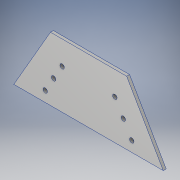
# Autodesk Inventor part: nhk22
Saved by Autodesk Inventor 2019 (Build 230136000, 136)
## iProperties
Created: 2022-02-15
Part Number: nhk22
Material: アルミニウム 6061
Document SubType Name: Sheet Metal
Designer: yuta
Density: 2.7 g/cm^3
Sheet Metal Rule: Default_mm
Appearance: アルミニウム - フラット
Author: yuta
Autodesk Inventor part; units mm, degrees
ref_plane "YZ Plane" through (0, 0, 0) normal (1, 0, 0) x (0, 1, 0)
ref_plane "XZ Plane" through (0, 0, 0) normal (0, 1, 0) x (-1, 0, 0)
ref_plane "XY Plane" through (0, 0, 0) normal (0, 0, 1) x (1, 0, 0)
sketch "スケッチ1" plane through (0, 0, 0) normal (0, 0, 1) x (1, 0, 0)
  line L0 (-21.0154, -61.075) -> (70.9846, -61.075)
  line L1 (70.9846, -61.075) -> (50.9846, -26.434)
  line L2 (50.9846, -26.434) -> (-1.0154, -26.434)
  line L3 (-1.0154, -26.434) -> (-21.0154, -61.075)
  point P0 (0, 0)
  dimension "d0" = 92
  dimension "d1" = 40
  dimension "d2" = 60
  dimension "d3" = 52
  constraints: 8 end point, 1 horizontal, 1 parallel
  measures "d0" distance of L0.start L0.end
  measures "d1" distance of L0.end L1.end
  measures "d2" angle of L1 L0
  measures "d3" distance of L1.end L2.end
extrude "押し出し1" add sketch "スケッチ1" along normal blind 2
sketch "スケッチ2" plane through (0, 0, 2) normal (0, 0, 1) x (1, 0, 0)
  circle A0 centre (6.975, -42.5942) radius 1.5
  line L0 (-1.0154, -26.434) -> (-21.0154, -61.075) projected
  line L1 (50.9846, -26.434) -> (-1.0154, -26.434) projected
  line L2 (-1.0154, -26.434) -> (24.9653, -41.434)
  line L3 (-1.0154, -26.434) -> (28.9846, -26.434) construction
  line L4 (70.9846, -61.075) -> (50.9846, -26.434) projected
  line L5 (50.9846, -26.434) -> (24.9751, -41.4506)
  circle A1 centre (1.2015, -52.5942) radius 1.5
  circle A2 centre (-4.572, -62.5942) radius 1.5
  line L6 (-21.0154, -61.075) -> (70.9846, -61.075) projected
  line L7 (-21.0154, -61.075) -> (-26.0154, -69.7352)
  line L8 (-21.0154, -61.075) -> (-11.0154, -61.075) construction
  line L9 (-26.0154, -69.7352) -> (75.9846, -69.7352)
  line L10 (75.9846, -69.7352) -> (70.9846, -61.075)
  point P0 (0, 0)
  dimension "d6" = 3
  dimension "d7" = 15
  dimension "d8" = 30
  dimension "d9" = 30
  dimension "d10" = 10
  dimension "d11" = 3
  dimension "d12" = 3
  dimension "d13" = 10
  dimension "d14" = 15
  dimension "d15" = 10
  dimension "d16" = 120
  dimension "d17" = 60
  dimension "d18" = 10
  dimension "d19" = 15
  constraints: 14 end point, 3 centre point, 2 equal length, 2 horizontal, 1 collinear, 1 perpendicular
  measures "d6" diameter of A0
  measures "d7" distance from line of L0 A0.centre
  measures "d8" distance of L0.start L2.end
  measures "d9" angle of L2 L3
  measures "d10" distance from line of L2 A0.centre
  measures "d11" diameter of A1
  measures "d12" diameter of A2
  measures "d13" vertical distance of A0.centre A1.centre
  measures "d14" distance from line of L0 A1.centre
  measures "d15" distance of L0.end L7.end
  measures "d16" angle of L7 L8
  measures "d17" angle of L9 L7
  measures "d18" vertical distance of A1.centre A2.centre
  measures "d19" distance from line of L0 A2.centre
extrude "押し出し2" add sketch "スケッチ2" against normal blind 2 contours L6 L10 L9 L7
sketch "スケッチ3" plane through (0, 0, 2) normal (0, 0, 1) x (1, 0, 0)
  line L0 (-1.0154, -26.434) -> (-26.0154, -69.7352) projected
  line L1 (-1.0154, -26.434) -> (24.9653, -41.434)
  line L2 (-1.0154, -26.434) -> (28.9846, -26.434) construction
  line L3 (24.9653, -41.434) -> (50.9461, -26.434)
  circle A0 centre (6.975, -42.5942) radius 1.5
  circle A1 centre (1.2015, -52.5942) radius 1.5
  circle A2 centre (42.9846, -42.5776) radius 1.5
  circle A3 centre (48.7581, -52.5776) radius 1.5
  circle A4 centre (54.5316, -62.5776) radius 1.5
  line L4 (75.9846, -69.7352) -> (50.9846, -26.434) projected
  point P0 (0, 0)
  dimension "d22" = 30
  dimension "d23" = 30
  dimension "d24" = 120
  dimension "d25" = 3
  dimension "d26" = 15
  dimension "d27" = 10
  dimension "d28" = 3
  dimension "d29" = 15
  dimension "d30" = 10
  dimension "d31" = 3
  dimension "d32" = 3
  dimension "d33" = 3
  dimension "d34" = 15
  dimension "d35" = 15
  dimension "d36" = 15
  dimension "d37" = 10
  dimension "d38" = 10
  dimension "d39" = 10
  constraints: 6 end point, 5 centre point, 1 equal length, 1 horizontal, 1 perpendicular
  measures "d22" distance of L0.start L1.end
  measures "d23" angle of L1 L2
  measures "d24" angle of L3 L1
  measures "d25" diameter of A0
  measures "d26" distance from line of L0 A0.centre
  measures "d27" distance from line of L1 A0.centre
  measures "d28" diameter of A1
  measures "d29" distance from line of L0 A1.centre
  measures "d30" vertical distance of A1.centre A0.centre
  measures "d31" diameter of A2
  measures "d32" diameter of A3
  measures "d33" diameter of A4
  measures "d34" distance from line of A2.centre L4
  measures "d35" distance from line of L4 A3.centre
  measures "d36" distance from line of L4 A4.centre
  measures "d37" distance from line of L3 A2.centre
  measures "d38" vertical distance of A3.centre A2.centre
  measures "d39" vertical distance of A4.centre A3.centre
hole "穴1" at (1.2015, -52.5942, 2) at (6.975, -42.5942, 2) at (42.9846, -42.5776, 2) at (54.5316, -62.5776, 2) at (48.7581, -52.5776, 2) direction (0, 0, -1) diameter 3 depth 2
equation "\"BendRadius\" = Thickness"
equation "\"BendReliefWidth\" = Thickness"
equation "\"BendReliefDepth\" = 0.5 * Thickness"
equation "\"CornerReliefSize\" = 4 * Thickness"
equation "\"MinimumRemnant\" = 2 * Thickness"
equation "\"TransitionRadius\" = BendRadius"
equation "\"JacobiRadiusSize\" = BendRadius"
equation "\"GapSize\" = Thickness"
equation "\"Thickness\" = 0.5"
